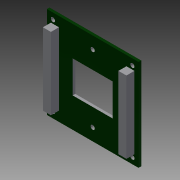
# Autodesk Inventor part: SFE-Host01
Saved by Autodesk Inventor 2015 (Build 190159000, 159)
## iProperties
Created: 2014-04-13
Part Number: SFE-Host01
Material: PCB(1)
Document SubType Name: Modeling
Designer: spichelh
Density: 1 g/cm^3
Appearance: Smooth - White(1)
Author: spichelh
Autodesk Inventor part; units mm, degrees
ref_plane "YZ Plane" through (0, 0, 0) normal (1, 0, 0) x (0, 1, 0)
ref_plane "XZ Plane" through (0, 0, 0) normal (0, 1, 0) x (-1, 0, 0)
ref_plane "XY Plane" through (0, 0, 0) normal (0, 0, 1) x (1, 0, 0)
sketch "Sketch1" plane through (0, 0, 0) normal (0, 0, 1) x (1, 0, 0)
  line L0 (-28.575, -28.575) -> (28.575, -28.575)
  line L1 (28.575, -28.575) -> (28.575, 28.575)
  line L2 (28.575, 28.575) -> (-28.575, 28.575)
  line L3 (-28.575, 28.575) -> (-28.575, -28.575)
  line L4 (-28.575, -28.575) -> (28.575, 28.575) construction
  line L5 (28.575, -28.575) -> (-28.575, 28.575) construction
  line L6 (-28.575, 0) -> (28.575, 0) construction
  line L7 (0, 28.575) -> (0, -28.575) construction
  circle A0 centre (-24.765, 24.765) radius 1.3
  circle A1 centre (24.765, 24.765) radius 1.3
  circle A2 centre (-24.765, -24.765) radius 1.3
  circle A3 centre (24.765, -24.765) radius 1.3
  circle A4 centre (0, -21) radius 1.3
  circle A5 centre (0, 21) radius 1.3
  line L8 (-12.5, 10) -> (12.5, 10)
  line L9 (12.5, 10) -> (12.5, -10)
  line L10 (12.5, -10) -> (-12.5, -10)
  line L11 (-12.5, -10) -> (-12.5, 10)
  line L12 (12.5, 10) -> (-12.5, -10) construction
  line L13 (12.5, -10) -> (-12.5, 10) construction
  point P0 (0, 0)
  point P1 (0, 0)
  dimension "d2" = 57.15
  dimension "d4" = 57.15
  dimension "d27" = 2.6
  dimension "d28" = 3.81
  dimension "d29" = 2.6
  dimension "d30" = 42
  dimension "d31" = 25
  dimension "d32" = 20
  constraints: 28 end point, 8 midpoint, 6 centre point, 4 parallel, 4 symmetric about line, 2 horizontal, 2 perpendicular, 2 point on line, 4 other
  measures "d2" distance of L1.end L2.end
  measures "d4" distance of L0.end L1.end
  measures "d27" diameter of A0
  measures "d28" distance from line of L2 A0.centre
  measures "d29" diameter of A4
  measures "d30" diameter of A4.centre L6
  measures "d31" distance of L8.start L8.end
  measures "d32" distance of L8.end L9.end
extrude "Extrusion1" add sketch "Sketch1" along normal blind 1.64
sketch "Sketch4" plane through (0, 0, 1.64) normal (0, 0, 1) x (1, 0, 0)
  line L0 (28.575, -28.575) -> (28.575, 28.575) projected
  line L1 (-28.575, 28.575) -> (-28.575, -28.575) projected
  line L2 (0, 0) -> (0, 45.0767)
  line L3 (21.035, 22.5) -> (26.035, 22.5)
  line L4 (26.035, 22.5) -> (26.035, -22.5)
  line L5 (26.035, -22.5) -> (21.035, -22.5)
  line L6 (21.035, -22.5) -> (21.035, 22.5)
  line L7 (-21.035, 22.5) -> (-26.035, 22.5)
  line L8 (-26.035, 22.5) -> (-26.035, -22.5)
  line L9 (-26.035, -22.5) -> (-21.035, -22.5)
  line L10 (-21.035, -22.5) -> (-21.035, 22.5)
  dimension "d21" = 2.54
  dimension "d22" = 45
  dimension "d23" = 5
  dimension "d24" = 22.5
  constraints: 18 end point, 4 symmetric about line, 3 parallel, 1 horizontal, 1 perpendicular
  measures "d21" distance between parallel lines of L4 L0
  measures "d22" distance between parallel lines of L5 L3
  measures "d23" distance between parallel lines of L4 L6
  measures "d24" distance from line of L2.start L3
extrude "Extrusion4" add sketch "Sketch4" along normal blind 5
body "Solid1"
